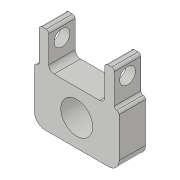
# Autodesk Inventor part: Needle Bearing Mount v2
Saved by Autodesk Inventor 2018.3 (Build 223284000, 284)
## iProperties
Created: 2019-03-08
Part Number: Needle Bearing Mount v2
Material: Generic
Document SubType Name: Modeling
Designer: aye06091
Mass: 23.7663 g
Surface Area: 78.4596 cm^2
Volume: 23.7663 cm^3
Density: 1 g/cm^3
Appearance: Default
Author: aye06091
Autodesk Inventor part; units mm, degrees
ref_plane "YZ Plane" through (0, 0, 0) normal (1, 0, 0) x (0, 1, 0)
ref_plane "XZ Plane" through (0, 0, 0) normal (0, 1, 0) x (-1, 0, 0)
ref_plane "XY Plane" through (0, 0, 0) normal (0, 0, 1) x (1, 0, 0)
sketch "Sketch1" plane through (0, 0, 0) normal (0, 0, 1) x (1, 0, 0)
  line L0 (0, 0) -> (50.8, 0)
  line L1 (50.8, 0) -> (50.8, -31.75)
  line L2 (50.8, -31.75) -> (0, -31.75)
  line L3 (0, -31.75) -> (0, 0)
  line L4 (2.8575, 0) -> (8.5725, 0)
  line L5 (8.5725, 0) -> (8.5725, 20.955)
  line L6 (8.5725, 20.955) -> (2.8575, 20.955)
  line L7 (2.8575, 20.955) -> (2.8575, 0)
  line L8 (42.2275, 0) -> (47.9425, 0)
  line L9 (47.9425, 0) -> (47.9425, 20.955)
  line L10 (47.9425, 20.955) -> (42.2275, 20.955)
  line L11 (42.2275, 20.955) -> (42.2275, 0)
  dimension "d1" = 31.75
  dimension "d4" = 5.715
  dimension "d5" = 5.715
  dimension "d21" = 20.955
  dimension "d32" = 50.8
  dimension "d35" = 2.8575
  dimension "d37" = 2.8575
  dimension "d38" = 33.655
  constraints: 24 end point, 6 parallel, 3 horizontal, 3 perpendicular, 3 point on line
  measures "d1" distance of L2.end L0.start
  measures "d4" distance between parallel lines of L9 L11
  measures "d5" distance of L5.end L6.end
  measures "d21" distance of L6.end L4.start
  measures "d32" distance between parallel lines of L1 L3
  measures "d35" distance between parallel lines of L3 L7
  measures "d37" distance between parallel lines of L1 L9
  measures "d38" distance between parallel lines of L11 L5
extrude "Extrusion1" add sketch "Sketch1" against normal blind 15.875
sketch "Sketch2" plane through (0, 0, 0) normal (0, 0, 1) x (1, 0, 0)
  circle A0 centre (25.4, -15.875) radius 9.5885
  line L0 (50.8, -31.75) -> (0, -31.75) projected
  line L1 (0, 0) -> (0, -31.75)
  dimension "d10" = 19.177
  dimension "d24" = 15.875
  dimension "d31" = 25.4
  constraints: 2 end point, 1 centre point, 1 vertical
  measures "d10" diameter of A0
  measures "d24" distance from line of L0 A0.centre
  measures "d31" distance from line of L1 A0.centre
extrude "Extrusion2" cut sketch "Sketch2" against normal through all
sketch "Sketch3" plane through (47.9425, 0, 0) normal (1, 0, 0) x (0, 0, -1)
  line L0 (0, 20.955) -> (15.875, 20.955) projected
  circle A0 centre (7.9375, 13.335) radius 4.7625
  dimension "d13" = 9.525
  dimension "d15" = 7.62
  constraints: 1 centre point
  measures "d13" diameter of A0
  measures "d15" distance from line of L0 A0.centre
extrude "Extrusion3" cut sketch "Sketch3" against normal up to next
fillet "Fillet2" radius 6.35 2 edges at (50.8, -31.75, -7.9375) (0, -31.75, -7.9375)
fillet "Fillet4" radius 1.5875 8 edges at (50.8, 0, -7.9375) (47.9425, 0, -7.9375) (47.9425, 20.955, -7.9375) (42.2275, 20.955, -7.9375) (8.5725, 20.955, -7.9375) (2.8575, 20.955, -7.9375) (0, 0, -7.9375) (2.8575, 0, -7.9375)
fillet "Fillet5" radius 3.175 2 edges at (8.5725, 0, -7.9375) (42.2275, 0, -7.9375)
sketch "Sketch4" plane through (8.5725, 19.3675, 0) normal (1, 0, 0) x (0, 0, -1)
  circle A0 centre (7.9375, -6.0325) radius 4.7625 projected
  circle A1 centre (7.9375, -6.0325) radius 4.7625
  point P0 (0, -19.3675)
  dimension "d26" = 9.525
  constraints: 1 centre point, 1 coincident
  measures "d26" diameter of A1
extrude "Extrusion4" cut sketch "Sketch4" against normal through all
body "Solid1"
